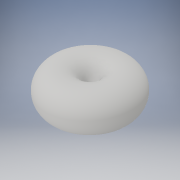
# Autodesk Inventor part: revloving donut
Saved by Autodesk Inventor 2017 (Build 210142000, 142)
## iProperties
Created: 2018-09-10
Part Number: revloving donut
Material: Generic
Document SubType Name: Modeling
Designer: qthuynh
Density: 1 g/cm^3
Appearance: Default
Author: qthuynh
Autodesk Inventor part; units mm, degrees
ref_plane "YZ Plane" through (0, 0, 0) normal (1, 0, 0) x (0, 1, 0)
ref_plane "XZ Plane" through (0, 0, 0) normal (0, 1, 0) x (-1, 0, 0)
ref_plane "XY Plane" through (0, 0, 0) normal (0, 0, 1) x (1, 0, 0)
sketch "Sketch1" plane through (0, 0, 0) normal (0, 0, 1) x (1, 0, 0)
  circle A0 centre (-5.0865, 3.9515) radius 17.2016
  line L0 (16.2264, -12.1488) -> (15.8481, 16.857)
  point P0 (0, 0)
  dimension "d0" = 360
  constraints: 2 end point, 1 centre point
revolve "Revolution1" add sketch "Sketch1" angle 360 about axis through (16.2264, -12.1488, 0) along (-0.013, 0.9999, 0)
body "Solid1"
